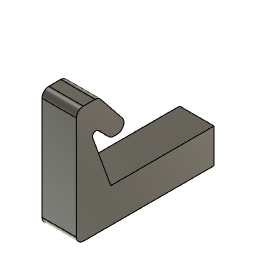
_HookM.3d233e70-de33-4639-a9dd-4a0a5d232dfa (Autodesk Fusion 360 design; units mm, degrees)
Autodesk Fusion 360 part; units mm, degrees
sketch "Sketch1" plane through (0, 0, 0) normal (1, 0, 0) x (0, 1, 0)
  line L0 (3.2, 17) -> (8, 11)
  line L1 (8, 11) -> (5, 11)
  line L2 (0, 17) -> (3.2, 17)
  line L3 (5, 11) -> (5, 5) construction
  line L4 (0, 17) -> (5, 9.0465) construction
  line L5 (20, 0) -> (0, 0)
  line L6 (5, 5) -> (1.5967, 14.4602)
  line L7 (0, 0) -> (0, 21) construction
  line L8 (0, 21) -> (8, 11) construction
  line L9 (5, 5) -> (20, 5)
  line L10 (0, 0) -> (0, 17)
  line L11 (1.5967, 14.4602) -> (5, 11)
  line L12 (2.1849, 12.8252) -> (2.8151, 13.2214) construction
  line L13 (20, 0) -> (20, 5)
  dimension "d4" = 20
  dimension "d5" = 8
  dimension "d6" = 5
  dimension "d7" = 21
  dimension "d8" = 6
  dimension "d9" = 5
  dimension "d25" = 17
  dimension "d26" = 3
  constraint perpendicular L5 L7
  constraint perpendicular L1 L7
  constraint perpendicular L1 L3
  constraint coincident L2.start L7
  constraint coincident L0.start L8
  constraint perpendicular L2 L7
  constraint coincident L4.end L3
  constraint coincident L6.end L4
  constraint coincident L12.start L6
  constraint coincident L12.end L11
  constraint perpendicular L4 L12
  constraint midpoint L4 L12
  constraint vertical L13
  constraint horizontal L9
  constraint horizontal L5
  constraint coincident L5.end L7.start
  measures "d4" distance of L5.start L5.end
  measures "d5" distance of L0.end L7
  measures "d6" distance of L3 L7
  measures "d7" distance of L7.end L5.end
  measures "d8" distance of L1.end L3.end
  measures "d9" distance of L5.start L9.end
  measures "d25" distance of L2 L5
  measures "d26" distance of L2.start L6.end
extrude "Extrude1" add sketch "Sketch1" along normal blind 5
fillet "Fillet1" radius 1 5 edges at (2.5, 3.2, 17) (2.5, 0, 17) (2.5, 0, 0) (2.5, 5, 11) (2.5, 8, 11)
fillet "Fillet2" radius 0.5 1 edges at (2.5, 1.5967, 14.4602)
